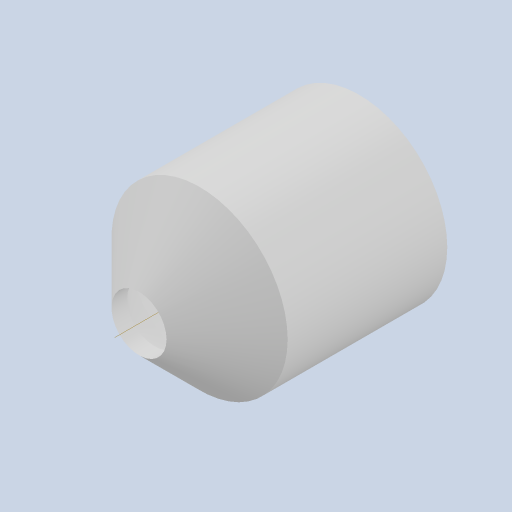
# Autodesk Inventor part: tapaimp
Saved by Autodesk Inventor 2023 (Build 270158000, 158)
## iProperties
Created: 2024-03-10
Part Number: tapaimp
Material: Generic
Document SubType Name: Modeling
Designer: dsone
Density: 1 g/cm^3
Appearance: Default
Author: dsone
Autodesk Inventor part; units mm, degrees
ref_plane "YZ Plane" through (0, 0, 0) normal (1, 0, 0) x (0, 1, 0)
ref_plane "XZ Plane" through (0, 0, 0) normal (0, 1, 0) x (-1, 0, 0)
ref_plane "XY Plane" through (0, 0, 0) normal (0, 0, 1) x (1, 0, 0)
sketch "Sketch1" plane through (0, 0, 0) normal (0, 0, 1) x (1, 0, 0)
  circle A0 centre (0, 0) radius 16
  dimension "d0" = 32
  constraints: 1 centre point, 1 coincident
  measures "d0" diameter of A0
extrude "Extrusion1" add sketch "Sketch1" along normal blind 40
chamfer "Chamfer1" distance 11 angle 45 1 edges at (-16, 0, 40)
shell "Shell1" thickness 2 removed faces 1 at (4.7224, 2.4785, 0)
sketch "Sketch2" plane through (0, 0, 40) normal (0, 0, 1) x (1, 0, 0)
  circle A0 centre (0, 0) radius 5 projected
extrude "Extrusion2" cut sketch "Sketch2" against normal blind 40
sketch "Sketch3" plane through (0, 0, 0) normal (1, 0, 0) x (0, 1, 0)
  line L0 (14, 0) -> (14, 28.1716) projected
  line L1 (14, 0) -> (-14, 0) projected
  line L2 (12.6679, -1.5) -> (14.4, -0.5)
  line L3 (14.4, -0.5) -> (14.4, -2.5)
  line L4 (14.4, -2.5) -> (12.6679, -1.5)
  point P0 (0, 0)
  point P1 (13.8226, -1.5)
  dimension "d9" = 2
  dimension "d10" = 0.4
  dimension "d11" = 0.5
  constraints: 6 end point, 1 vertical, 7 other
  measures "d9" distance of L2.end L3.end
  measures "d10" distance from line of L0 L2.end
  measures "d11" distance from line of L1 L2.end
coil "Coil1" sketch "Sketch3" operation add axis through (0, 0, 0) along (0, 0, 1) pitch 2 turns 10.5 hand right
sketch "Sketch4" plane through (0, 0, 0) normal (0, 0, -1) x (-1, 0, 0)
  circle A0 centre (0, 0) radius 15.1002
  constraints: 1 centre point, 1 coincident
extrude "Extrusion3" cut sketch "Sketch4" along normal blind 40
sketch "Sketch5" plane through (0, -14, 20.2691) normal (1, 0, 0) x (0, 0, -1)
  point P0 (20.2691, 14)
body "Solid1"
